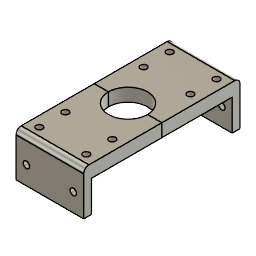
_Other Rotating Bracket.333db4ca-e624-4356-8ae1-39af13bcdd5d (Autodesk Fusion 360 design; units mm, degrees)
Autodesk Fusion 360 part; units mm, degrees
note: some values were not read from the file. Set by a fixed rule: which sketch regions a step uses.
sketch "Sketch1" plane through (0, 0, 0) normal (0, 1, 0) x (1, 0, 0)
  line L0 (0, 0) -> (26, 0)
  line L1 (26, 0) -> (26, -30)
  line L2 (26, -30) -> (0, -30)
  line L3 (0, -30) -> (0, 0)
  circle A0 centre (13, 0) radius 7.5
  circle A1 centre (22, -15) radius 1.25
  circle A2 centre (22, -25) radius 1.25
  circle A3 centre (4, -15) radius 1.25
  circle A4 centre (4, -25) radius 1.25
  dimension "d16" = 26
  dimension "d17" = 30
  dimension "d18" = 15
  dimension "d19" = 2.5
  dimension "d20" = 2.5
  dimension "d21" = 2.5
  dimension "d22" = 2.5
  dimension "d23" = 5
  dimension "d24" = 10
  dimension "d25" = 5
  dimension "d26" = 10
  dimension "d27" = 4
  dimension "d28" = 4
  dimension "d29" = 4
  dimension "d30" = 4
  constraint horizontal L0
  constraint vertical L1
  constraint horizontal L2
  constraint vertical L3
  constraint coincident L0.start L3.end
  constraint midpoint L0 A0.centre
  measures "d16" distance of L0.start L0.end
  measures "d17" distance of L0.start L2.end
  measures "d18" diameter of A0
  measures "d19" diameter of A1
  measures "d20" diameter of A2
  measures "d21" diameter of A3
  measures "d22" diameter of A4
  measures "d23" distance of L2 A4.centre
  measures "d24" vertical distance of A3.centre A4.centre
  measures "d25" distance of L2 A2.centre
  measures "d26" vertical distance of A1.centre A2.centre
  measures "d27" distance of L1 A1.centre
  measures "d28" distance of L1 A2.centre
  measures "d29" distance of L3 A3.centre
  measures "d30" distance of L3 A4.centre
extrude "Extrude1" add sketch "Sketch1" along normal blind 5 contours L0 L1 L2 L3 A0 makes body 1
sketch "Sketch2" plane through (0, 0, 0) normal (0, -1, 0) x (1, 0, 0)
  circle A0 centre (4, 15) radius 1.25
  circle A1 centre (22, 25) radius 1.25
  circle A2 centre (4, 25) radius 1.25
  circle A3 centre (22, 15) radius 1.25
  line L0 (0, 30) -> (0, 0)
  line L1 (0, 0) -> (5.5, 0)
  arc A4 (20.5, 0) -> (5.5, 0) centre (13, 0) ccw
  line L2 (20.5, 0) -> (26, 0)
  line L3 (26, 0) -> (26, 30)
  line L4 (26, 30) -> (0, 30)
  line L5 (26, 30) -> (0, 30)
  line L6 (0, 30) -> (0, 27)
  line L7 (0, 27) -> (26, 27)
  line L8 (26, 27) -> (26, 30)
  constraint horizontal L5
  constraint vertical L6
  constraint horizontal L7
  constraint vertical L8
  constraint coincident L0 L6.end
  constraint coincident L3.end L4.start
extrude "Extrude2" add sketch "Sketch2" along normal blind 12 contours L0 L3 L4 L5 L6 L7 L8 bodies 1
sketch "Sketch3" plane through (0, 0, 30) normal (0, 0, 1) x (1, 0, 0)
  line L0 (26, -12) -> (26, 5)
  line L1 (26, 5) -> (0, 5)
  line L2 (0, 5) -> (0, -12)
  line L3 (0, -12) -> (26, -12)
  circle A0 centre (4, -5) radius 1.25
  circle A1 centre (22, -5) radius 1.25
  dimension "d35" = 2.5
  dimension "d36" = 2.5
  dimension "d37" = 4
  dimension "d38" = 4
  dimension "d39" = 10
  dimension "d40" = 10
  measures "d35" diameter of A0
  measures "d36" diameter of A1
  measures "d37" distance of L2 A0.centre
  measures "d38" distance of L0 A1.centre
  measures "d39" distance of L1 A0.centre
  measures "d40" distance of L1 A1.centre
extrude "Extrude3" cut sketch "Sketch3" against normal blind 6 contours A0 | A1 bodies 1
ref_plane "WorkPlane1" through (26, 0, 0) normal (0, 0, -1) x (-1, 0, 0)
mirror "Mirror1" about plane through (26, 0, 0) normal (0, 0, -1) of bodies 1 makes body 2
fillet "Fillet1" radius 2 1 edges at (13, 5, -30) on bodies 2
fillet "Fillet2" radius 2 1 edges at (13, 5, 30) on bodies 1
